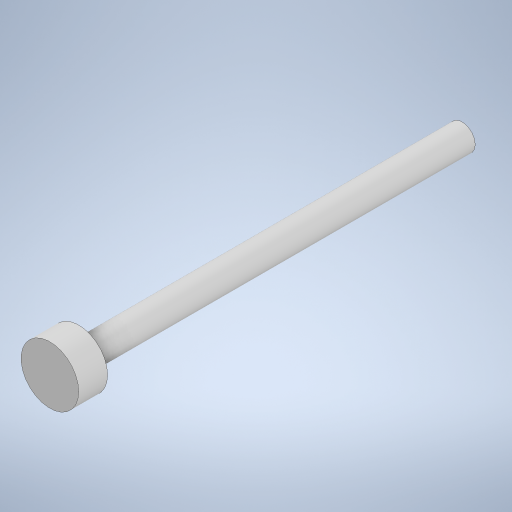
# Autodesk Inventor part: rod_130mm
Saved by Autodesk Inventor 2023 (Build 270158000, 158)
## iProperties
Created: 2023-02-11
Part Number: rod_130mm
Material: Generic
Document SubType Name: Modeling
Designer: Nikhil
Density: 1 g/cm^3
Appearance: Default
Author: Nikhil
Autodesk Inventor part; units mm, degrees
ref_plane "YZ Plane" through (0, 0, 0) normal (1, 0, 0) x (0, 1, 0)
ref_plane "XZ Plane" through (0, 0, 0) normal (0, 1, 0) x (-1, 0, 0)
ref_plane "XY Plane" through (0, 0, 0) normal (0, 0, 1) x (1, 0, 0)
sketch "Sketch1" plane through (0, 0, 0) normal (0, 0, 1) x (1, 0, 0)
  circle A0 centre (0, 0) radius 6.35
  dimension "d0" = 12.7
  constraints: 1 centre point, 1 coincident
  measures "d0" diameter of A0
extrude "Extrusion1" add sketch "Sketch1" along normal blind 200
sketch "Sketch2" plane through (0, 0, 200) normal (0, 0, 1) x (1, 0, 0)
  circle A0 centre (0, 0) radius 6.35 projected
  circle A1 centre (0, 0) radius 14
  dimension "d3" = 28
  constraints: 1 centre point, 1 coincident
  measures "d3" diameter of A1
extrude "Extrusion2" add sketch "Sketch2" against normal blind 14
body "Solid1"
